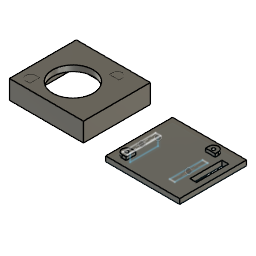
Joystick Rig pt4_ (Autodesk Fusion 360 design; units mm, degrees)
part number: 2026-02-06-13-37-08-094
Autodesk Fusion 360 part; units mm, degrees
note: some values were not read from the file. Set by a fixed rule: which sketch regions a step uses.
sketch "Sketch3" plane through (0, 0, 0) normal (0, 0, 1) x (1, 0, 0)
  line L0 (0, 0) -> (16.95, 0)
  line L1 (16.95, 0) -> (16.95, 19)
  line L2 (16.95, 19) -> (0, 19)
  line L3 (0, 19) -> (0, 0)
  circle A0 centre (8, 9.3) radius 8
  circle A1 centre (14.6, 20.25) radius 0.8
  circle A2 centre (14.6, 20.25) radius 1.9
  line L4 (16.5, 20.25) -> (12.7, 20.25)
  line L5 (12.7, 20.25) -> (12.7, 19)
  line L6 (12.7, 19) -> (16.5, 19)
  line L7 (16.5, 19) -> (16.5, 20.25)
  circle A3 centre (-1.6, 2.2) radius 0.725
  circle A4 centre (-1.6, 2.2) radius 1.9
  line L8 (0, 4.1) -> (0, 0)
  line L9 (-1.6, 0.3) -> (0, 0.3)
  line L10 (0, 0.3) -> (0, 4.1)
  line L11 (0, 4.1) -> (-1.6, 4.1)
  line L12 (-1.6, 4.1) -> (-1.6, 0.3)
  line L13 (21.45, 19.3) -> (18.85, 19.3)
  line L14 (18.85, 19.3) -> (18.85, 16.7)
  line L15 (18.85, 16.7) -> (21.45, 16.7)
  line L16 (21.45, 16.7) -> (21.45, 19.3)
  line L17 (21.45, 19.3) -> (18.85, 16.7) construction
  line L18 (18.85, 19.3) -> (21.45, 16.7) construction
  line L19 (18.85, 19.3) -> (21.45, 19.3)
  line L20 (21.45, 19.3) -> (21.45, 6.7)
  line L21 (21.45, 6.7) -> (18.85, 6.7)
  line L22 (18.85, 6.7) -> (18.85, 19.3)
  circle A5 centre (52.6, 20.25) radius 1.9
  line L23 (38, 4.1) -> (38, 0)
  line L24 (59.45, 6.7) -> (56.85, 6.7)
  line L25 (50.7, 19) -> (54.5, 19)
  line L26 (59.45, 19.3) -> (56.85, 19.3)
  circle A6 centre (36.4, 2.2) radius 0.725
  line L27 (36.4, 0.3) -> (38, 0.3)
  line L28 (54.5, 19) -> (54.5, 20.25)
  line L29 (56.85, 19.3) -> (59.45, 19.3)
  line L30 (56.85, 6.7) -> (56.85, 19.3)
  line L31 (38, 0.3) -> (38, 4.1)
  circle A7 centre (52.6, 20.25) radius 0.8
  line L32 (36.4, 4.1) -> (36.4, 0.3)
  line L33 (54.95, 0) -> (54.95, 19)
  line L34 (56.85, 19.3) -> (56.85, 16.7)
  line L35 (59.45, 19.3) -> (59.45, 6.7)
  line L36 (59.45, 19.3) -> (56.85, 16.7) construction
  line L37 (54.95, 19) -> (38, 19)
  circle A8 centre (36.4, 2.2) radius 1.9
  line L38 (38, 4.1) -> (36.4, 4.1)
  line L39 (56.85, 19.3) -> (59.45, 16.7) construction
  line L40 (54.5, 20.25) -> (50.7, 20.25)
  line L41 (56.85, 16.7) -> (59.45, 16.7)
  line L42 (38, 0) -> (54.95, 0)
  line L43 (59.45, 16.7) -> (59.45, 19.3)
  circle A9 centre (46, 9.3) radius 8
  line L44 (50.7, 20.25) -> (50.7, 19)
  line L45 (38, 19) -> (38, 0)
  point P0 (8, 9.3)
  point P1 (14.6, 20.25)
  point P2 (-1.6, 2.2)
  point P3 (20.15, 18)
  point P4 (20.15, 18)
  point P5 (38, 0)
  point P6 (52.6, 20.25)
  point P7 (46, 9.3)
  point P8 (36.4, 2.2)
  point P9 (58.15, 18)
  point P10 (58.15, 18)
  dimension "d8" = 16.95
  dimension "d9" = 19
  dimension "d10" = 9.3
  dimension "d11" = 8
  dimension "d12" = 16
  dimension "d13" = 10.95
  dimension "d14" = 14.6
  dimension "d15" = 1.6
  dimension "d16" = 3.8
  dimension "d17" = 7.1
  dimension "d18" = 16.2
  dimension "d19" = 1.45
  dimension "d20" = 3.8
  dimension "d21" = 5.55
  dimension "d22" = 2.25
  dimension "d23" = 2.6
  dimension "d24" = 2.6
  dimension "d25" = 2.6
  dimension "d26" = 12.6
  dimension "d40" = 16.95
  dimension "d41" = 19
  dimension "d42" = 9.3
  dimension "d43" = 8
  dimension "d44" = 16
  dimension "d45" = 10.95
  dimension "d46" = 14.6
  dimension "d47" = 1.6
  dimension "d48" = 3.8
  dimension "d49" = 7.1
  dimension "d50" = 16.2
  dimension "d51" = 1.45
  dimension "d52" = 3.8
  dimension "d53" = 5.55
  dimension "d54" = 2.25
  dimension "d55" = 2.6
  dimension "d56" = 2.6
  dimension "d57" = 2.6
  dimension "d58" = 12.6
  constraint horizontal L0
  constraint vertical L1
  constraint horizontal L2
  constraint vertical L3
  constraint coincident L0.start L3.end
  constraint coincident P0 A0.centre
  constraint coincident P1 A1.centre
  constraint horizontal L4
  constraint vertical L5
  constraint horizontal L6
  constraint vertical L7
  constraint coincident L2 L5.end
  constraint coincident A2 L4.start
  constraint coincident P2 A3.centre
  constraint concentric A3 A4
  constraint vertical L8
  constraint horizontal L9
  constraint vertical L10
  constraint horizontal L11
  constraint vertical L12
  constraint coincident A4 L9.start
  constraint horizontal L13
  constraint perpendicular L13 L14
  constraint parallel L13 L15
  constraint parallel L14 L16
  constraint coincident L17 P4
  constraint coincident L18 P4
  constraint coincident P4 P3
  constraint horizontal L19
  constraint vertical L20
  constraint horizontal L21
  constraint vertical L22
  constraint horizontal L42
  constraint vertical L33
  constraint horizontal L37
  constraint vertical L45
  constraint coincident P5 L23.end
  constraint coincident P7 A9.centre
  constraint coincident P6 A5.centre
  constraint horizontal L40
  constraint vertical L44
  constraint horizontal L25
  constraint vertical L28
  constraint coincident L25.start L37
  constraint coincident L28.end A5
  constraint coincident P8 A6.centre
  constraint concentric A6 A8
  constraint vertical L23
  constraint horizontal L27
  constraint vertical L31
  constraint horizontal L38
  constraint vertical L32
  constraint coincident L27.start A8
  constraint horizontal L26
  constraint perpendicular L26 L34
  constraint parallel L26 L41
  constraint parallel L34 L43
  constraint coincident P10 L36
  constraint coincident P10 L39
  constraint coincident P10 P9
  constraint horizontal L29
  constraint vertical L35
  constraint horizontal L24
  constraint vertical L30
  measures "d8" distance of L0.start L0.end
  measures "d9" distance of L0.start L2.end
  measures "d10" distance of L0 P0
  measures "d11" distance of L3 P0
  measures "d12" diameter of A0
  measures "d13" vertical distance of P0 P1
  measures "d14" distance of L3 P1
  measures "d15" diameter of A1
  measures "d16" diameter of A2
  measures "d17" vertical distance of P0 P2
  measures "d18" horizontal distance of P1 P2
  measures "d19" diameter of A3
  measures "d20" diameter of A4
  measures "d21" horizontal distance of P1 P4
  measures "d22" vertical distance of P1 P4
  measures "d23" distance of L14.end L15.end
  measures "d24" distance of L13.end L14.end
  measures "d25" distance of L13.end L13.start
  measures "d26" distance of L13.end L21.end
  measures "d40" distance of P5 L33.start
  measures "d41" distance of P5 L37.end
  measures "d42" distance of P7 L42
  measures "d43" distance of P7 L45
  measures "d44" diameter of A9
  measures "d45" vertical distance of P6 P7
  measures "d46" distance of P6 L45
  measures "d47" diameter of A7
  measures "d48" diameter of A5
  measures "d49" vertical distance of P7 P8
  measures "d50" horizontal distance of P8 P6
  measures "d51" diameter of A6
  measures "d52" diameter of A8
  measures "d53" horizontal distance of P6 P10
  measures "d54" vertical distance of P6 P10
  measures "d55" distance of L39.end L34.end
  measures "d56" distance of L26.end L34.end
  measures "d57" distance of L26.end L26.start
  measures "d58" distance of L26.end L24.end
sketch "Sketch5" plane through (0, 0, 0) normal (0, 0, 1) x (1, 0, 0)
  line L0 (21.65, 22.25) -> (-3.6, 22.25)
  line L1 (-3.6, 22.25) -> (-3.6, -0.2)
  line L2 (-3.6, -0.2) -> (21.65, -0.2)
  line L3 (21.65, -0.2) -> (21.65, 22.25)
  line L4 (21.45, 19.3) -> (21.45, 6.7)
  line L5 (0, 0) -> (16.95, 0)
  line L6 (-5.6, -2.2) -> (23.65, -2.2)
  line L7 (23.65, -2.2) -> (23.65, 24.25)
  line L8 (23.65, 24.25) -> (-5.6, 24.25)
  line L9 (-5.6, 24.25) -> (-5.6, -2.2)
  line L10 (61.65, 24.25) -> (32.4, 24.25)
  line L11 (34.4, -0.2) -> (59.65, -0.2)
  line L12 (38, 0) -> (54.95, 0)
  line L13 (32.4, 24.25) -> (32.4, -2.2)
  line L14 (32.4, -2.2) -> (61.65, -2.2)
  line L15 (61.65, -2.2) -> (61.65, 24.25)
  line L16 (59.65, 22.25) -> (34.4, 22.25)
  line L17 (34.4, 22.25) -> (34.4, -0.2)
  line L18 (59.45, 19.3) -> (59.45, 6.7)
  line L19 (59.65, -0.2) -> (59.65, 22.25)
  point P0 (-1.6, 2.2)
  point P1 (14.6, 20.25)
  point P2 (38, 0)
  point P3 (36.4, 2.2)
  point P4 (52.6, 20.25)
  dimension "d28" = 2
  dimension "d29" = 2
  dimension "d30" = 0.2
  dimension "d31" = 0.2
  dimension "d32" = 2
  dimension "d33" = 2
  dimension "d34" = 2
  dimension "d35" = 2
  dimension "d69" = 2
  dimension "d70" = 2
  dimension "d71" = 0.2
  dimension "d72" = 0.2
  dimension "d73" = 2
  dimension "d74" = 2
  dimension "d75" = 2
  dimension "d76" = 2
  constraint horizontal L0
  constraint vertical L1
  constraint horizontal L2
  constraint vertical L3
  constraint horizontal L6
  constraint vertical L7
  constraint horizontal L8
  constraint vertical L9
  constraint horizontal L16
  constraint vertical L17
  constraint horizontal L11
  constraint vertical L19
  constraint horizontal L14
  constraint vertical L15
  constraint horizontal L10
  constraint vertical L13
  measures "d28" distance of L1 P0
  measures "d29" distance of L0 P1
  measures "d30" distance of L3 L4
  measures "d31" distance of L2 L5
  measures "d32" distance of L2 L6
  measures "d33" distance of L3 L7
  measures "d34" distance of L1 L9
  measures "d35" distance of L0 L8
  measures "d69" distance of P3 L17
  measures "d70" distance of P4 L16
  measures "d71" distance of L18 L19
  measures "d72" distance of L11 L12
  measures "d73" distance of L11 L14
  measures "d74" distance of L15 L19
  measures "d75" distance of L13 L17
  measures "d76" distance of L10 L16
extrude "Extrude3" add sketch "Sketch5" along normal blind 7.5 contours L0 L1 L2 L3 | L6 L7 L8 L9 makes body 1
extrude "Extrude4" cut sketch "Sketch5" along normal blind 5.2 contours L0 L1 L2 L3 bodies 1
extrude "Extrude5" cut sketch "Sketch3" along normal blind 8 contours A0 bodies 1
extrude "Extrude6" add sketch "Sketch3" along normal blind 7.2 separate body contours L3 A4 L8 L9 L10 | L3 A3 A4 L8 L10 L12 | A3 A4 L12 | L2 A2 L6 L7 | L3 A4 L8 L10 L11 | A3 L12 | A3 L12 | L2 A1 A2 L4 L6 | A1 A2 L4 | L2 A2 L5 L6 | A1 L4 | A1 L4 makes body 2 at (-1.6947, 0.3024, 4.8) makes body 3 at (12.7094, 20.4392, 2.4)
extrude "Extrude7" cut sketch "Sketch3" along normal blind 2.45 contours L3 A4 L8 L9 L10 | L3 A3 A4 L8 L10 L12 | A3 A4 L12 | L2 A2 L6 L7 | L3 A4 L8 L10 L11 | A3 L12 | A3 L12 | L2 A1 A2 L4 L6 | A1 A2 L4 | L2 A2 L5 L6 | A1 L4 | A1 L4 bodies 2 3
extrude "Extrude8" add sketch "Sketch3" sketch "Sketch5" against normal blind 2 separate body contours A5 A7 L40 | A5 L25 L28 L37 | A5 L25 A7 L37 L40 | A5 L25 L37 L44 | A9 | A5 L23 L25 L31 L33 L37 A8 L42 L45 | A5 L25 L37 | A7 L40 | A7 L40 | L23 L31 A8 L38 L45 | L23 L27 L31 A8 L45 | L23 L31 A8 L45 | L23 A6 L31 L32 A8 L45 | A6 L32 A8 | A6 L32 | A6 L32 | L24 L30 L35 L41 | L26 L29 L30 L34 L35 L41 L43 of sketch 2 contours L10 L13 L14 L15 | L11 L16 L17 L19 makes body 4
extrude "Extrude9" cut sketch "Sketch3" against normal blind 2 contours L24 L30 L35 L41 | L26 L29 L30 L34 L35 L41 L43 bodies 4
extrude "Extrude10" add sketch "Sketch3" along normal blind 1.2 contours A5 A7 L40 | A5 L25 L28 L37 | A5 L25 A7 L37 L40 | A5 L25 L37 L44 | A7 L40 | A7 L40 | L23 L31 A8 L38 L45 | L23 L27 L31 A8 L45 | L23 A6 L31 L32 A8 L45 | A6 L32 A8 | A6 L32 | A6 L32 bodies 4
sketch "Sketch9" plane through (0, 0, -2) normal (0, 0, -1) x (1, 0, 0)
  line L0 (59.45, -19.3) -> (56.85, -19.3)
  line L1 (56.85, -19.3) -> (56.85, -6.7)
  line L2 (56.85, -6.7) -> (59.45, -6.7)
  line L3 (59.45, -6.7) -> (59.45, -19.3)
  line L4 (61.65, -24.25) -> (61.65, 2.2)
  line L5 (61.65, 2.2) -> (32.4, 2.2)
  line L6 (32.4, 2.2) -> (32.4, -24.25)
  line L7 (32.4, -24.25) -> (61.65, -24.25)
  line L8 (54.95, 0) -> (54.95, -19)
  circle A0 centre (52.6, -20.25) radius 0.8
  line L9 (21.45, -6.7) -> (18.85, -6.7)
  line L10 (-1.6, -0.3) -> (0, -0.3)
  circle A1 centre (36.4, -2.2) radius 0.725
  line L11 (50.7, -20.25) -> (50.7, -19)
  line L12 (59.45, -16.7) -> (59.45, -19.3)
  line L13 (18.85, -19.3) -> (21.45, -16.7) construction
  line L14 (56.85, -19.3) -> (59.45, -19.3)
  line L15 (21.45, -19.3) -> (21.45, -6.7)
  line L16 (56.85, -19.3) -> (59.45, -16.7) construction
  line L17 (0, -0.3) -> (0, -4.1)
  line L18 (16.95, -19) -> (0, -19)
  line L19 (12.7, -19) -> (16.5, -19)
  circle A2 centre (36.4, -2.2) radius 1.9
  line L20 (0, -19) -> (0, 0)
  line L21 (36.4, -4.1) -> (36.4, -0.3)
  line L22 (38, 0) -> (54.95, 0)
  line L23 (36.4, -0.3) -> (38, -0.3)
  circle A3 centre (-1.6, -2.2) radius 1.9
  line L24 (12.7, -20.25) -> (12.7, -19)
  line L25 (38, -19) -> (38, 0)
  line L26 (18.85, -19.3) -> (18.85, -16.7)
  line L27 (0, 0) -> (16.95, 0)
  line L28 (18.85, -6.7) -> (18.85, -19.3)
  line L29 (59.45, -6.7) -> (56.85, -6.7)
  line L30 (21.45, -16.7) -> (21.45, -19.3)
  circle A4 centre (8, -9.3) radius 8
  line L31 (56.85, -19.3) -> (56.85, -16.7)
  circle A5 centre (52.6, -20.25) radius 1.9
  line L32 (56.85, -6.7) -> (56.85, -19.3)
  line L33 (18.85, -16.7) -> (21.45, -16.7)
  line L34 (0, -4.1) -> (-1.6, -4.1)
  line L35 (18.85, -19.3) -> (21.45, -19.3)
  circle A6 centre (46, -9.3) radius 8
  line L36 (54.5, -20.25) -> (50.7, -20.25)
  line L37 (0, -4.1) -> (0, 0)
  circle A7 centre (14.6, -20.25) radius 1.9
  line L38 (59.45, -19.3) -> (59.45, -6.7)
  line L39 (38, -4.1) -> (36.4, -4.1)
  line L40 (38, -0.3) -> (38, -4.1)
  line L41 (16.5, -19) -> (16.5, -20.25)
  line L42 (50.7, -19) -> (54.5, -19)
  line L43 (38, -4.1) -> (38, 0)
  line L44 (21.45, -19.3) -> (18.85, -16.7) construction
  line L45 (16.5, -20.25) -> (12.7, -20.25)
  line L46 (21.45, -19.3) -> (18.85, -19.3)
  line L47 (56.85, -16.7) -> (59.45, -16.7)
  line L48 (-1.6, -4.1) -> (-1.6, -0.3)
  line L49 (54.5, -19) -> (54.5, -20.25)
  line L50 (54.95, -19) -> (38, -19)
  circle A8 centre (-1.6, -2.2) radius 0.725
  line L51 (59.45, -19.3) -> (56.85, -19.3)
  circle A9 centre (14.6, -20.25) radius 0.8
  line L52 (16.95, 0) -> (16.95, -19)
  line L53 (59.45, -19.3) -> (56.85, -16.7) construction
  point P0 (14.6, -20.25)
  point P1 (20.15, -18)
  point P2 (8, -9.3)
  point P3 (38, 0)
  point P4 (20.15, -18)
  point P5 (58.15, -18)
  point P6 (52.6, -20.25)
  point P7 (46, -9.3)
  point P8 (36.4, -2.2)
  point P9 (-1.6, -2.2)
  point P10 (58.15, -18)
  dimension "d85" = 16.95
  dimension "d86" = 19
  dimension "d87" = 9.3
  dimension "d88" = 8
  dimension "d89" = 16
  dimension "d91" = 14.6
  dimension "d92" = 1.6
  dimension "d93" = 3.8
  dimension "d96" = 1.45
  dimension "d97" = 3.8
  dimension "d100" = 2.6
  dimension "d101" = 2.6
  dimension "d102" = 2.6
  dimension "d103" = 12.6
  dimension "d104" = 16.95
  dimension "d105" = 19
  dimension "d106" = 9.3
  dimension "d107" = 8
  dimension "d108" = 16
  dimension "d110" = 14.6
  dimension "d111" = 1.6
  dimension "d112" = 3.8
  dimension "d115" = 1.45
  dimension "d116" = 3.8
  dimension "d119" = 2.6
  dimension "d120" = 2.6
  dimension "d121" = 2.6
  dimension "d122" = 12.6
  constraint coincident L20.end L27.start
  constraint coincident P2 A4.centre
  constraint coincident P0 A7.centre
  constraint coincident L19.start L18
  constraint coincident L41.end A7
  constraint coincident P9 A3.centre
  constraint concentric A3 A8
  constraint coincident L10.start A3
  constraint perpendicular L26 L46
  constraint parallel L33 L46
  constraint parallel L26 L30
  constraint coincident P4 L44
  constraint coincident P4 L13
  constraint coincident P4 P1
  constraint coincident P3 L22.start
  constraint coincident P7 A6.centre
  constraint coincident P6 A0.centre
  constraint coincident L11.end L50
  constraint coincident L36.start A5
  constraint coincident P8 A1.centre
  constraint concentric A1 A2
  constraint coincident L21.end A2
  constraint perpendicular L31 L51
  constraint parallel L47 L51
  constraint parallel L12 L31
  constraint coincident P10 L53
  constraint coincident P10 L16
  constraint coincident P10 P5
  measures "d85" distance of L20.end L27.end
  measures "d86" distance of L20.end L18.end
  measures "d87" distance of P2 L27
  measures "d88" distance of P2 L20
  measures "d89" diameter of A4
  measures "d91" distance of P0 L20
  measures "d92" diameter of A9
  measures "d93" diameter of A7
  measures "d96" diameter of A8
  measures "d97" diameter of A3
  measures "d100" distance of L26.end L13.end
  measures "d101" distance of L26.end L13.start
  measures "d102" distance of L13.start L15.start
  measures "d103" distance of L13.start L9.end
  measures "d104" distance of L8.start P3
  measures "d105" distance of P3 L25.start
  measures "d106" distance of P7 L22
  measures "d107" distance of P7 L25
  measures "d108" diameter of A6
  measures "d110" distance of P6 L25
  measures "d111" diameter of A0
  measures "d112" diameter of A5
  measures "d115" diameter of A1
  measures "d116" diameter of A2
  measures "d119" distance of L31.end L12.start
  measures "d120" distance of L0.end L31.end
  measures "d121" distance of L0.end L0.start
  measures "d122" distance of L0.end L1.end
hole "Hole1" at (52.6, 20.25, -2) at (36.4, 2.2, -2) at (14.6, 20.25, -2) at (-1.6, 2.2, -2) direction (0, 0, 1) diameter 1.271 depth 7 tip angle 180 counterbore diameter 3 counterbore depth 1 bodies 2 3 4
thread "Thread1" "ISO Metric profile 1.6 M1.6x0.35 M1.6x0.35 6H" thread offset 0 thread depth 7.4
sketch "Sketch10" plane through (0, 0, -2) normal (0, 0, -1) x (1, 0, 0)
  circle A0 centre (52.6, -20.25) radius 1.5
  circle A1 centre (36.4, -2.2) radius 1.5
  line L0 (59.45, -19.3) -> (56.85, -19.3)
  line L1 (56.85, -19.3) -> (56.85, -6.7)
  line L2 (56.85, -6.7) -> (59.45, -6.7)
  line L3 (59.45, -6.7) -> (59.45, -19.3)
  line L4 (61.65, -24.25) -> (61.65, 2.2)
  line L5 (61.65, 2.2) -> (32.4, 2.2)
  line L6 (32.4, 2.2) -> (32.4, -24.25)
  line L7 (32.4, -24.25) -> (61.65, -24.25)
  line L8 (34.4, -4.525) -> (32.4, -4.525)
  line L9 (32.4, -4.525) -> (32.4, -17.525)
  line L10 (32.4, -17.525) -> (34.4, -17.525)
  line L11 (34.4, -17.525) -> (34.4, -4.525)
  line L12 (34.4, -4.525) -> (32.4, -17.525) construction
  line L13 (32.4, -4.525) -> (34.4, -17.525) construction
  line L14 (51, -17.525) -> (53, -17.525)
  line L15 (53, -17.525) -> (53, -4.525)
  line L16 (53, -4.525) -> (51, -4.525)
  line L17 (51, -4.525) -> (51, -17.525)
  line L18 (51, -17.525) -> (53, -4.525) construction
  line L19 (53, -17.525) -> (51, -4.525) construction
  point P0 (33.4, -11.025)
  point P1 (52, -11.025)
  dimension "d130" = 2
  dimension "d131" = 13
  dimension "d132" = 2
  dimension "d133" = 13
  constraint horizontal L8
  constraint perpendicular L8 L9
  constraint parallel L8 L10
  constraint parallel L9 L11
  constraint coincident L12 P0
  constraint coincident L13 P0
  constraint midpoint L6 L9
  constraint horizontal L14
  constraint perpendicular L14 L15
  constraint parallel L14 L16
  constraint parallel L15 L17
  constraint coincident L18 P1
  constraint coincident L19 P1
  constraint collinear L10 L14
  measures "d130" distance of L9.end L10.end
  measures "d131" distance of L8.end L9.end
  measures "d132" distance of L15.end L16.end
  measures "d133" distance of L14.end L15.end
extrude "Extrude11" add sketch "Sketch10" along normal blind 4 contours L6 L8 L9 L10 L11 | L14 L15 L16 L17 bodies 4
sketch "Sketch11" plane through (34.4, 0, 0) normal (1, 0, 0) x (0, 1, 0)
  line L0 (17.525, -2) -> (4.525, -2)
  line L1 (4.525, -2) -> (4.525, -6)
  line L2 (4.525, -6) -> (17.525, -6)
  line L3 (17.525, -6) -> (17.525, -2)
  line L4 (16.5, -2) -> (5.5, -2)
  line L5 (5.5, -2) -> (5.5, -5)
  line L6 (5.5, -5) -> (16.5, -5)
  line L7 (16.5, -5) -> (16.5, -2)
  dimension "d136" = 11
  constraint horizontal L4
  constraint vertical L5
  constraint horizontal L6
  constraint vertical L7
  constraint coincident L0 L4.start
  measures "d136" distance of L4.start L4.end
extrude "Extrude12" cut sketch "Sketch11" against normal blind 2 contours L0 L4 L5 L6 L7 bodies 4
extrude "Extrude13" cut sketch "Sketch11" along normal blind 19 contours L0 L4 L5 L6 L7 bodies 4
